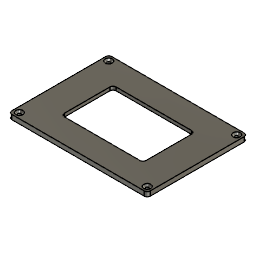
Lid V3.4 (Autodesk Fusion 360 design; units mm, degrees)
part number: 2026-01-29-14-58-12-979
Autodesk Fusion 360 part; units mm, degrees
note: some values were not read from the file. Set by a fixed rule: which sketch regions a step uses.
sketch "Sketch2" plane through (0, 0, 0) normal (0, 0, 1) x (1, 0, 0)
  line L0 (-48, 52) -> (124, 52)
  line L1 (128, 48) -> (128, -74)
  line L2 (124, -78) -> (-48, -78)
  line L3 (-52, -74) -> (-52, 48)
  circle A0 centre (-45, 45) radius 2.25
  line L4 (38, -78) -> (38, 52) construction
  line L5 (-52, -13) -> (128, -13) construction
  arc A1 (-48, 52) -> (-52, 48) centre (-48, 48) ccw
  circle A2 centre (121, 45) radius 2.25
  arc A3 (128, 48) -> (124, 52) centre (124, 48) ccw
  circle A4 centre (121, -71) radius 2.25
  arc A5 (124, -78) -> (128, -74) centre (124, -74) ccw
  circle A6 centre (-45, -71) radius 2.25
  arc A7 (-52, -74) -> (-48, -78) centre (-48, -74) ccw
  point P0 (-52, 52)
  point P1 (128, 52)
  dimension "d3" = 4.5
  dimension "d4" = 7
  dimension "d5" = 7
  dimension "d6" = 4
  dimension "d63" = 180
  dimension "d64" = 130
  constraint horizontal L0
  constraint vertical L1
  constraint horizontal L2
  constraint vertical L3
  constraint coincident L0 L4.end
  constraint coincident L3 L5.start
  constraint coincident P0 L0
  constraint coincident P0 L3
  constraint tangent L0 A1
  constraint tangent L3 A1
  constraint symmetric P0 L4 P1
  constraint symmetric A0 L4 A2
  constraint symmetric L4 L0.start L0.end
  constraint symmetric L4 L3.end L1.start
  constraint symmetric L4 A1 A3
  constraint coincident L1 L5.end
  constraint symmetric A0 L5 A6
  constraint symmetric L5 L0.start L2.end
  constraint symmetric L5 L3.end L3.start
  constraint symmetric L5 A1 A7
  constraint symmetric L5 L1.start L1.end
  constraint symmetric L5 L0.end L2.start
  constraint symmetric L5 A2 A4
  constraint symmetric L5 A3 A5
  constraint coincident L2 L4.start
  measures "d3" diameter of A0
  measures "d4" distance of L0 A0.centre
  measures "d5" distance of L3 A0.centre
  measures "d6" radius of A1
  measures "d63" distance of L1 L3
  measures "d64" distance of L0 L2
extrude "Extrude1" add sketch "Sketch2" along normal blind 6
sketch "Sketch3" plane through (0, 0, 0) normal (0, 0, -1) x (1, 0, 0)
  circle A0 centre (121, 71) radius 2.25
  circle A1 centre (-45, 71) radius 2.25
  circle A2 centre (-45, -45) radius 2.25
  circle A3 centre (121, -45) radius 2.25
  arc A4 (-52, -48) -> (-48, -52) centre (-48, -48) ccw
  line L0 (-48, -52) -> (124, -52)
  arc A5 (124, -52) -> (128, -48) centre (124, -48) ccw
  line L1 (128, -48) -> (128, 74)
  arc A6 (128, 74) -> (124, 78) centre (124, 74) ccw
  line L2 (124, 78) -> (-48, 78)
  arc A7 (-48, 78) -> (-52, 74) centre (-48, 74) ccw
  line L3 (-52, 74) -> (-52, -48)
  line L4 (38, 78) -> (38, -52) construction
  line L5 (128, 13) -> (-52, 13) construction
  line L6 (117.9494, -41.9494) -> (-41.9494, -41.9494) construction
  line L7 (-41.9494, -41.9494) -> (-41.9494, 67.9494) construction
  line L8 (-41.9494, 67.9494) -> (117.9494, 67.9494) construction
  line L9 (117.9494, 67.9494) -> (117.9494, -41.9494) construction
  line L10 (117.9494, -41.9494) -> (-41.9494, 67.9494) construction
  line L11 (-41.9494, -41.9494) -> (117.9494, 67.9494) construction
  line L12 (106.2459, -44.0839) -> (-30.2459, -44.0839)
  line L13 (-44.0839, -30.2459) -> (-44.0839, 56.2459)
  line L14 (-30.2459, 70.0839) -> (106.2459, 70.0839)
  line L15 (120.0839, 56.2459) -> (120.0839, -30.2459)
  line L16 (93.976, -25.9276) -> (-44.0839, 70.0839) construction
  line L17 (-38.2879, -33.8258) -> (83.9414, 41.199) construction
  line L18 (-39.8149, -30.2459) -> (-39.8149, 56.2459)
  line L19 (-30.2459, 65.8149) -> (106.2459, 65.8149)
  line L20 (115.8149, 56.2459) -> (115.8149, -30.2459)
  line L21 (103.0391, -31.1436) -> (-39.8149, 65.8149) construction
  line L22 (-35.6113, -30.989) -> (81.1607, 38.7921) construction
  arc A8 (-30.2459, 65.8149) -> (-39.8149, 56.2459) centre (-30.2459, 56.2459) ccw
  arc A9 (-30.2459, 70.0839) -> (-44.0839, 56.2459) centre (-30.2459, 56.2459) ccw
  arc A10 (115.8149, 56.2459) -> (106.2459, 65.8149) centre (106.2459, 56.2459) ccw
  arc A11 (120.0839, 56.2459) -> (106.2459, 70.0839) centre (106.2459, 56.2459) ccw
  arc A12 (-39.8149, -30.2459) -> (-30.2459, -39.8149) centre (-30.2459, -30.2459) ccw
  arc A13 (-44.0839, -30.2459) -> (-30.2459, -44.0839) centre (-30.2459, -30.2459) ccw
  arc A14 (106.2459, -39.8149) -> (115.8149, -30.2459) centre (106.2459, -30.2459) ccw
  arc A15 (106.2459, -44.0839) -> (120.0839, -30.2459) centre (106.2459, -30.2459) ccw
  line L23 (106.2459, -39.8149) -> (-30.2459, -39.8149)
  point P0 (38, 13)
  point P1 (38, 13)
  point P2 (38, 13)
  point P3 (38, 13)
  point P4 (38, 13)
  dimension "d25" = 159.8988
  dimension "d27" = 109.8988
  dimension "d28" = 2.1345
  dimension "d29" = 2.1345
  dimension "d30" = 2.1345
  dimension "d31" = 2.1345
  dimension "d44" = 9.569
  dimension "d45" = 13.838
  constraint midpoint L2 L4.start
  constraint midpoint L0 L4.end
  constraint midpoint L1 L5.start
  constraint midpoint L3 L5.end
  constraint midpoint L4 P4
  constraint coincident P4 P3
  constraint horizontal L6
  constraint perpendicular L6 L7
  constraint parallel L6 L8
  constraint parallel L7 L9
  constraint coincident L10 P4
  constraint coincident L11 P4
  constraint horizontal L12
  constraint perpendicular L12 L13
  constraint parallel L12 L14
  constraint parallel L13 L15
  constraint coincident L16 P4
  constraint coincident L17 P4
  constraint perpendicular L18 L23
  constraint parallel L19 L23
  constraint parallel L18 L20
  constraint coincident L21 P4
  constraint coincident L22 P4
  constraint coincident L21.end L19
  constraint coincident L21.end L18
  constraint tangent L19 A8
  constraint tangent L18 A8
  constraint coincident L16.end L14
  constraint coincident L16.end L13
  constraint tangent L14 A9
  constraint tangent L13 A9
  constraint symmetric L4 L19.start L19.end
  constraint symmetric L4 L18.end L20.start
  constraint symmetric L4 A8 A10
  constraint symmetric L4 L14.start L14.end
  constraint symmetric L4 L13.end L15.start
  constraint symmetric L4 A9 A11
  constraint symmetric L5 L19.start A12.end
  constraint symmetric L5 L18.end L18.start
  constraint symmetric L5 A8 A12
  constraint symmetric L5 L14.start L12.end
  constraint symmetric L5 L13.end L13.start
  constraint symmetric L5 A9 A13
  constraint symmetric L5 L19.end A14.start
  constraint symmetric L5 L20.start L20.end
  constraint symmetric L5 A10 A14
  constraint symmetric L5 L14.end L12.start
  constraint symmetric L5 L15.start L15.end
  constraint symmetric L5 A11 A15
  measures "d25" distance of L7.end L8.end
  measures "d27" distance of L6.end L7.end
  measures "d28" distance of L9 L15
  measures "d29" distance of L8 L14
  measures "d30" distance of L8 L19
  measures "d31" distance of L9 L20
  measures "d44" radius of A8
  measures "d45" radius of A9
extrude "Extrude4" add sketch "Sketch3" along normal blind 1.424 contours L12 L13 L14 L15 A9 A11 A13 A15
draft "Draft3" angle 10 neutral plane through (0, 0, -1.424) pull (0, 0, -1) 16 faces at (60.7486, -65.8149, -0.9493) (109.3756, -65.2886, -0.9493) (115.8149, -27.4153, -0.4747) (108.5019, 39.5452, -0.9493) (60.7486, 39.8149, -0.4747) (-38.5329, 35.0304, -0.9493) (-39.8149, -27.4153, -0.4747) (-32.5019, -65.5452, -0.9493) (-44.0839, 1.4153, -0.4747) (-35.389, 43.0927, -0.9493) (15.2514, 44.0839, -0.9493) (116.2609, 39.7952, -0.9493) (120.0839, 1.4153, -0.9493) (108.8648, -69.8338, -0.9493) (60.7486, -70.0839, -0.9493) (-44.0213, -57.5613, -0.4747)
sketch "Sketch5" plane through (0, 0, -1.424) normal (0, 0, -1) x (1, 0, 0)
  line L0 (-30.2459, 65.8149) -> (106.2459, 65.8149)
  line L1 (115.8149, 56.2459) -> (115.8149, -30.2459)
  line L2 (106.2459, -39.8149) -> (-30.2459, -39.8149)
  line L3 (-39.8149, -30.2459) -> (-39.8149, 56.2459)
  line L4 (106.2459, 70.0839) -> (-30.2459, 70.0839)
  line L5 (-44.0839, 56.2459) -> (-44.0839, -30.2459)
  line L6 (-30.2459, -44.0839) -> (106.2459, -44.0839)
  line L7 (120.0839, -30.2459) -> (120.0839, 56.2459)
  line L8 (38, 70.0839) -> (38, -44.0839) construction
  line L9 (120.0839, 13) -> (-44.0839, 13) construction
  line L10 (117.9494, -41.9494) -> (-41.9494, -41.9494) construction
  line L11 (-41.9494, -41.9494) -> (-41.9494, 67.9494) construction
  line L12 (-41.9494, 67.9494) -> (117.9494, 67.9494) construction
  line L13 (117.9494, 67.9494) -> (117.9494, -41.9494) construction
  line L14 (117.9494, -41.9494) -> (-41.9494, 67.9494) construction
  line L15 (-41.9494, -41.9494) -> (117.9494, 67.9494) construction
  line L16 (106.2459, -42.8839) -> (-30.2459, -42.8839)
  line L17 (-42.8839, -30.2459) -> (-42.8839, 56.2459)
  line L18 (-30.2459, 68.8839) -> (106.2459, 68.8839)
  line L19 (118.8839, 56.2459) -> (118.8839, -30.2459)
  line L20 (96.0985, -27.1411) -> (-42.8839, 68.8839) construction
  line L21 (-42.8839, -42.8839) -> (96.0985, 53.1411) construction
  line L22 (106.2459, -41.0149) -> (-30.2459, -41.0149)
  line L23 (-41.0149, -30.2459) -> (-41.0149, 56.2459)
  line L24 (117.0149, 56.2459) -> (117.0149, -30.2459)
  line L25 (95.1479, -26.0666) -> (-41.0149, 67.0149) construction
  line L26 (-41.0149, -41.0149) -> (95.1479, 52.0666) construction
  arc A0 (115.8149, 56.2459) -> (106.2459, 65.8149) centre (106.2459, 56.2459) ccw
  arc A1 (106.2459, -39.8149) -> (115.8149, -30.2459) centre (106.2459, -30.2459) ccw
  arc A2 (-39.8149, -30.2459) -> (-30.2459, -39.8149) centre (-30.2459, -30.2459) ccw
  arc A3 (-30.2459, 65.8149) -> (-39.8149, 56.2459) centre (-30.2459, 56.2459) ccw
  arc A4 (-44.0839, -30.2459) -> (-30.2459, -44.0839) centre (-30.2459, -30.2459) ccw
  arc A5 (106.2459, -44.0839) -> (120.0839, -30.2459) centre (106.2459, -30.2459) ccw
  arc A6 (120.0839, 56.2459) -> (106.2459, 70.0839) centre (106.2459, 56.2459) ccw
  arc A7 (-30.2459, 70.0839) -> (-44.0839, 56.2459) centre (-30.2459, 56.2459) ccw
  arc A8 (-30.2459, 67.0149) -> (-41.0149, 56.2459) centre (-30.2459, 56.2459) ccw
  arc A9 (-30.2459, 68.8839) -> (-42.8839, 56.2459) centre (-30.2459, 56.2459) ccw
  arc A10 (117.0149, 56.2459) -> (106.2459, 67.0149) centre (106.2459, 56.2459) ccw
  arc A11 (118.8839, 56.2459) -> (106.2459, 68.8839) centre (106.2459, 56.2459) ccw
  line L27 (-30.2459, 67.0149) -> (106.2459, 67.0149)
  arc A12 (106.2459, -41.0149) -> (117.0149, -30.2459) centre (106.2459, -30.2459) ccw
  arc A13 (106.2459, -42.8839) -> (118.8839, -30.2459) centre (106.2459, -30.2459) ccw
  arc A14 (-41.0149, -30.2459) -> (-30.2459, -41.0149) centre (-30.2459, -30.2459) ccw
  arc A15 (-42.8839, -30.2459) -> (-30.2459, -42.8839) centre (-30.2459, -30.2459) ccw
  point P0 (38, 13)
  point P1 (38, 13)
  point P2 (38, 13)
  dimension "d36" = 159.8988
  dimension "d37" = 109.8988
  dimension "d38" = 0.9345
  dimension "d39" = 0.9345
  dimension "d40" = 0.9345
  dimension "d41" = 0.9345
  dimension "d50" = 10.769
  dimension "d51" = 12.638
  constraint midpoint L4 L8.start
  constraint midpoint L6 L8.end
  constraint midpoint L7 L9.start
  constraint midpoint L5 L9.end
  constraint horizontal L10
  constraint perpendicular L10 L11
  constraint parallel L10 L12
  constraint parallel L11 L13
  constraint coincident L14 P2
  constraint coincident L15 P2
  constraint midpoint L8 P2
  constraint horizontal L16
  constraint perpendicular L16 L17
  constraint parallel L16 L18
  constraint parallel L17 L19
  constraint coincident L20 P2
  constraint coincident L21 P2
  constraint coincident P2 P1
  constraint horizontal L22
  constraint perpendicular L22 L23
  constraint parallel L22 L27
  constraint parallel L23 L24
  constraint coincident L25 P2
  constraint coincident L26 P2
  constraint coincident L26.start L23
  constraint coincident L26.start L22
  constraint coincident L21.start L17
  constraint coincident L21.start L16
  constraint coincident L25.end L27
  constraint coincident L25.end L23
  constraint tangent A8 L27
  constraint tangent L23 A8
  constraint coincident L20.end L18
  constraint coincident L20.end L17
  constraint tangent L18 A9
  constraint tangent L17 A9
  constraint symmetric L8 A8.start A10.end
  constraint symmetric L8 L23.end L24.start
  constraint symmetric L8 A8 A10
  constraint symmetric L8 L18.start L18.end
  constraint symmetric L8 L17.end L19.start
  constraint symmetric L8 A9 A11
  constraint symmetric L9 A10.end L22.start
  constraint symmetric L9 L24.start L24.end
  constraint symmetric L9 A10 A12
  constraint symmetric L9 L18.end L16.start
  constraint symmetric L9 L19.start L19.end
  constraint symmetric L9 A11 A13
  constraint symmetric L9 A8.start L22.end
  constraint symmetric L9 L23.end L23.start
  constraint symmetric L9 A8 A14
  constraint symmetric L9 L18.start L16.end
  constraint symmetric L9 L17.end L17.start
  constraint symmetric L9 A9 A15
  constraint coincident L23.start A14.start
  constraint coincident L17.start A15.start
  constraint coincident L22.end A14.end
  constraint coincident L16.end A15.end
  measures "d36" distance of L11.end L12.end
  measures "d37" distance of L10.end L11.end
  measures "d38" distance of L13 L19
  measures "d39" distance of L13 L24
  measures "d40" distance of L10 L16
  measures "d41" distance of L10 L22
  measures "d50" radius of A8
  measures "d51" radius of A9
extrude "Extrude6" cut sketch "Sketch5" against normal blind 1.424 contours L16 L17 L18 L19 A9 A11 A13 A15
extrude "Extrude7" cut 1 faces at (15.2514, -30.5213, 0) along direction (0, 0, 1) blind 0.5
sketch "Sketch6" plane through (0, 0, 0.5) normal (0, 0, -1) x (1, 0, 0)
  line L0 (106.2459, 65.5638) -> (-30.2459, 65.5638)
  arc A0 (-30.2459, 65.5638) -> (-39.5638, 56.2459) centre (-30.2459, 56.2459) ccw
  line L1 (-39.5638, 56.2459) -> (-39.5638, -30.2459)
  arc A1 (-39.5638, -30.2459) -> (-30.2459, -39.5638) centre (-30.2459, -30.2459) ccw
  line L2 (-30.2459, -39.5638) -> (106.2459, -39.5638)
  arc A2 (106.2459, -39.5638) -> (115.5638, -30.2459) centre (106.2459, -30.2459) ccw
  line L3 (115.5638, -30.2459) -> (115.5638, 56.2459)
  arc A3 (115.5638, 56.2459) -> (106.2459, 65.5638) centre (106.2459, 56.2459) ccw
  line L4 (38, 65.5638) -> (38, -39.5638) construction
  line L5 (-39.5638, 13) -> (115.5638, 13) construction
  line L6 (92, -25.5) -> (-16, -25.5)
  line L7 (-20, -21.5) -> (-20, 47.5)
  line L8 (-16, 51.5) -> (92, 51.5)
  line L9 (96, 47.5) -> (96, -21.5)
  line L10 (96, -25.5) -> (-20, 51.5) construction
  line L11 (-20, -25.5) -> (96, 51.5) construction
  arc A4 (-16, 51.5) -> (-20, 47.5) centre (-16, 47.5) ccw
  arc A5 (96, 47.5) -> (92, 51.5) centre (92, 47.5) ccw
  arc A6 (92, -25.5) -> (96, -21.5) centre (92, -21.5) ccw
  arc A7 (-20, -21.5) -> (-16, -25.5) centre (-16, -21.5) ccw
  point P0 (38, 13)
  dimension "d58" = 116
  dimension "d59" = 77
  dimension "d68" = 4
  dimension "d69" = 4
  dimension "d70" = 4
  dimension "d71" = 4
  constraint midpoint L0 L4.start
  constraint midpoint L2 L4.end
  constraint midpoint L1 L5.start
  constraint midpoint L3 L5.end
  constraint horizontal L6
  constraint perpendicular L6 L7
  constraint parallel L6 L8
  constraint parallel L7 L9
  constraint coincident L10 P0
  constraint coincident L11 P0
  constraint midpoint L5 P0
  constraint coincident L10.end L8
  constraint coincident L10.end L7
  constraint tangent L8 A4
  constraint tangent L7 A4
  constraint coincident L11.end L8
  constraint coincident L11.end L9
  constraint tangent L8 A5
  constraint tangent L9 A5
  constraint coincident L10.start L9
  constraint coincident L10.start L6
  constraint tangent L9 A6
  constraint tangent L6 A6
  constraint coincident L11.start L7
  constraint coincident L11.start L6
  constraint tangent L7 A7
  constraint tangent L6 A7
  measures "d58" distance of L10.end L11.end
  measures "d59" distance of L11.start L10.end
  measures "d68" radius of A4
  measures "d69" radius of A5
  measures "d70" radius of A6
  measures "d71" radius of A7
extrude "Extrude8" cut sketch "Sketch6" against normal blind 1.1 contours L6 L7 L8 L9 A4 A5 A6 A7
sketch "Sketch7" plane through (0, 0, 1.6) normal (0, 0, -1) x (1, 0, 0)
  line L0 (92, 51.5) -> (-16, 51.5)
  line L1 (-20, 47.5) -> (-20, -21.5)
  line L2 (-16, -25.5) -> (92, -25.5)
  line L3 (96, -21.5) -> (96, 47.5)
  line L4 (38, 51.5) -> (38, -25.5) construction
  line L5 (96, 13) -> (-20, 13) construction
  line L6 (87, -20.5) -> (-11, -20.5)
  line L7 (-15, -16.5) -> (-15, 42.5)
  line L8 (-11, 46.5) -> (87, 46.5)
  line L9 (91, 42.5) -> (91, -16.5)
  line L10 (91, -20.5) -> (-15, 46.5) construction
  line L11 (-15, -20.5) -> (91, 46.5) construction
  arc A0 (-16, 51.5) -> (-20, 47.5) centre (-16, 47.5) ccw
  arc A1 (-20, -21.5) -> (-16, -25.5) centre (-16, -21.5) ccw
  arc A2 (92, -25.5) -> (96, -21.5) centre (92, -21.5) ccw
  arc A3 (96, 47.5) -> (92, 51.5) centre (92, 47.5) ccw
  arc A4 (-11, 46.5) -> (-15, 42.5) centre (-11, 42.5) ccw
  arc A5 (91, 42.5) -> (87, 46.5) centre (87, 42.5) ccw
  arc A6 (87, -20.5) -> (91, -16.5) centre (87, -16.5) ccw
  arc A7 (-15, -16.5) -> (-11, -20.5) centre (-11, -16.5) ccw
  point P0 (38, 13)
  dimension "d62" = 106
  dimension "d65" = 67
  dimension "d72" = 4
  dimension "d73" = 4
  dimension "d74" = 4
  dimension "d75" = 4
  constraint midpoint L0 L4.start
  constraint midpoint L2 L4.end
  constraint midpoint L3 L5.start
  constraint midpoint L1 L5.end
  constraint horizontal L6
  constraint perpendicular L6 L7
  constraint parallel L6 L8
  constraint parallel L7 L9
  constraint coincident L10 P0
  constraint coincident L11 P0
  constraint midpoint L4 P0
  constraint coincident L10.end L8
  constraint coincident L10.end L7
  constraint tangent L8 A4
  constraint tangent L7 A4
  constraint coincident L11.end L9
  constraint coincident L11.end L8
  constraint tangent L9 A5
  constraint tangent L8 A5
  constraint coincident L10.start L9
  constraint coincident L10.start L6
  constraint tangent L9 A6
  constraint tangent L6 A6
  constraint coincident L11.start L6
  constraint coincident L11.start L7
  constraint tangent L6 A7
  constraint tangent L7 A7
  measures "d62" distance of L10.end L11.end
  measures "d65" distance of L11.start L10.end
  measures "d72" radius of A4
  measures "d73" radius of A5
  measures "d74" radius of A6
  measures "d75" radius of A7
extrude "Extrude9" cut sketch "Sketch7" against normal blind 8.4 contours L6 L7 L8 L9 A4 A5 A6 A7
sketch "Sketch9" plane through (0, 0, 6) normal (0, 0, 1) x (-1, 0, 0)
  line L0 (15, 42.5) -> (15, -16.5)
  arc A0 (11, -20.5) -> (15, -16.5) centre (11, -16.5) ccw
  line L1 (11, -20.5) -> (-87, -20.5)
  arc A1 (-91, -16.5) -> (-87, -20.5) centre (-87, -16.5) ccw
  line L2 (-91, -16.5) -> (-91, 42.5)
  arc A2 (-87, 46.5) -> (-91, 42.5) centre (-87, 42.5) ccw
  line L3 (-87, 46.5) -> (11, 46.5)
  arc A3 (15, 42.5) -> (11, 46.5) centre (11, 42.5) ccw
  circle A4 centre (-121, 71) radius 2.25
  circle A5 centre (-121, -45) radius 2.25
  circle A6 centre (45, 71) radius 2.25
  circle A7 centre (45, -45) radius 2.25
  arc A8 (48, -52) -> (52, -48) centre (48, -48) ccw
  line L4 (52, -48) -> (52, 74)
  arc A9 (52, 74) -> (48, 78) centre (48, 74) ccw
  line L5 (48, 78) -> (-124, 78)
  arc A10 (-124, 78) -> (-128, 74) centre (-124, 74) ccw
  line L6 (-128, 74) -> (-128, -48)
  arc A11 (-128, -48) -> (-124, -52) centre (-124, -48) ccw
  line L7 (-124, -52) -> (48, -52)
  line L8 (45, -47.25) -> (45, -42.75) construction
  line L9 (42.75, -45) -> (47.25, -45) construction
  circle A12 centre (45, -45) radius 4
  line L10 (-38, -52) -> (-38, 78) construction
  line L11 (-128, 13) -> (52, 13) construction
  circle A13 centre (-121, -45) radius 4
  circle A14 centre (45, 71) radius 4
  circle A15 centre (-121, 71) radius 4
  dimension "d91" = 8
  constraint coincident A7 L8.start
  constraint coincident A7 L8.end
  constraint vertical L8
  constraint coincident A7 L9.start
  constraint coincident A7 L9.end
  constraint perpendicular L8 L9
  constraint concentric A7 A12
  constraint midpoint L7 L10.start
  constraint midpoint L5 L10.end
  constraint midpoint L6 L11.start
  constraint midpoint L4 L11.end
  constraint symmetric A12 L10 A13
  constraint symmetric A12 L11 A14
  constraint symmetric L11 A13 A15
  measures "d91" diameter of A12
sketch "Sketch10" plane through (0, 0, 0.5) normal (0, 0, -1) x (1, 0, 0)
  line L0 (-20, -21.5) -> (-20, 47.5)
  arc A0 (-16, 51.5) -> (-20, 47.5) centre (-16, 47.5) ccw
  line L1 (-16, 51.5) -> (92, 51.5)
  arc A1 (96, 47.5) -> (92, 51.5) centre (92, 47.5) ccw
  line L2 (96, 47.5) -> (96, -21.5)
  arc A2 (92, -25.5) -> (96, -21.5) centre (92, -21.5) ccw
  line L3 (92, -25.5) -> (-16, -25.5)
  arc A3 (-20, -21.5) -> (-16, -25.5) centre (-16, -21.5) ccw
  line L4 (106.2459, 65.5638) -> (-30.2459, 65.5638)
  arc A4 (-30.2459, 65.5638) -> (-39.5638, 56.2459) centre (-30.2459, 56.2459) ccw
  line L5 (-39.5638, 56.2459) -> (-39.5638, -30.2459)
  arc A5 (-39.5638, -30.2459) -> (-30.2459, -39.5638) centre (-30.2459, -30.2459) ccw
  line L6 (-30.2459, -39.5638) -> (106.2459, -39.5638)
  arc A6 (106.2459, -39.5638) -> (115.5638, -30.2459) centre (106.2459, -30.2459) ccw
  line L7 (115.5638, -30.2459) -> (115.5638, 56.2459)
  arc A7 (115.5638, 56.2459) -> (106.2459, 65.5638) centre (106.2459, 56.2459) ccw
  line L8 (38, 65.5638) -> (38, -39.5638) construction
  line L9 (115.5638, 13) -> (-39.5638, 13) construction
  line L10 (38, 13) -> (-24.24, 13) construction
  line L11 (-23.09, 11) -> (-25.39, 11)
  line L12 (-25.39, 11) -> (-25.39, 15)
  line L13 (-25.39, 15) -> (-23.09, 15)
  line L14 (-23.09, 15) -> (-23.09, 11)
  line L15 (-23.09, 11) -> (-25.39, 15) construction
  line L16 (-25.39, 11) -> (-23.09, 15) construction
  line L17 (38, 13) -> (38, 54) construction
  line L18 (40, 52.85) -> (36, 52.85)
  line L19 (36, 52.85) -> (36, 55.15)
  line L20 (36, 55.15) -> (40, 55.15)
  line L21 (40, 55.15) -> (40, 52.85)
  line L22 (40, 52.85) -> (36, 55.15) construction
  line L23 (36, 52.85) -> (40, 55.15) construction
  line L24 (99.09, 15) -> (99.09, 11)
  line L25 (101.39, 15) -> (99.09, 15)
  line L26 (101.39, 11) -> (101.39, 15)
  line L27 (99.09, 11) -> (101.39, 11)
  line L28 (40, -26.85) -> (36, -26.85)
  line L29 (40, -29.15) -> (40, -26.85)
  line L30 (36, -29.15) -> (40, -29.15)
  line L31 (36, -26.85) -> (36, -29.15)
  point P0 (-24.24, 13)
  point P1 (38, 54)
  dimension "d97" = 62.24
  dimension "d98" = 2.3
  dimension "d99" = 4
  dimension "d100" = 41
  dimension "d101" = 2.3
  dimension "d102" = 4
  constraint midpoint L4 L8.start
  constraint midpoint L6 L8.end
  constraint midpoint L7 L9.start
  constraint midpoint L5 L9.end
  constraint midpoint L9 L10.start
  constraint perpendicular L8 L10
  constraint horizontal L11
  constraint perpendicular L11 L12
  constraint parallel L11 L13
  constraint parallel L12 L14
  constraint coincident L15 P0
  constraint coincident L16 P0
  constraint coincident P0 L10.end
  constraint perpendicular L9 L17
  constraint horizontal L18
  constraint perpendicular L18 L19
  constraint parallel L18 L20
  constraint parallel L19 L21
  constraint coincident L22 P1
  constraint coincident L23 P1
  constraint coincident P1 L17.end
  constraint symmetric L8 L11.start L24.end
  constraint symmetric L8 L11.end L26.start
  constraint symmetric L8 L12.end L25.start
  constraint symmetric L8 L13.end L24.start
  constraint symmetric L9 L18.start L28.start
  constraint symmetric L9 L18.end L28.end
  constraint symmetric L9 L19.end L30.start
  constraint symmetric L9 L20.end L29.start
  measures "d97" distance of L10.start P0
  measures "d98" distance of L12.end L13.end
  measures "d99" distance of L11.end L12.end
  measures "d100" distance of L10.start P1
  measures "d101" distance of L18.start L20.end
  measures "d102" distance of L19.end L20.end
extrude "Extrude12" add sketch "Sketch10" along normal blind 4.2 contours L11 L12 L13 L14 | L18 L19 L20 L21 | L24 L25 L26 L27 | L28 L29 L30 L31
chamfer "Chamfer2" distance 2.4 angle 45 4 edges at (-47.0977, 45.8136, 6) (118.9023, 45.8136, 6) (118.9023, -70.1864, 6) (-47.0977, -70.1864, 6) measured on face at (111.574, -3.1667, 6) measured on face at (111.574, -3.1667, 6) measured on face at (111.574, -3.1667, 6) measured on face at (111.574, -3.1667, 6)
equation "d3 = Bolt_Diam + 0.5 mm"
equation "ORingDiameter = 1.78 mm" comment "Diamter of the O ring"
equation "ORingInnerDiameter = 170 mm" comment "Inner diamter of the o ring bore"
equation "d25 = ( ORingPerimeter - 100 mm ) / 4 + 50 mm"
equation "ORingPerimeter = 2 * 3.1412 * ( ( ORingInnerDiameter / 2 ) + ORingDiameter / 2 )"
equation "d27 = ( ORingPerimeter - 100 mm ) / 4"
equation "d28 = ( ( ORingDiameter * 1.05 ) / 2 ) + 1.2 mm"
equation "d29 = ( ( ORingDiameter * 1.05 ) / 2 ) + 1.2 mm"
equation "d30 = ( ( ORingDiameter * 1.05 ) / 2 ) + 1.2 mm"
equation "d31 = ( ( ORingDiameter * 1.05 ) / 2 ) + 1.2 mm"
equation "d32 = ORingDiameter * 0.8"
equation "d36 = ( ORingPerimeter - 100 mm ) / 4 + 50 mm"
equation "d37 = ( ORingPerimeter - 100 mm ) / 4"
equation "d38 = ( ORingDiameter * 1.05 ) / 2"
equation "d39 = ( ORingDiameter * 1.05 ) / 2"
equation "d40 = ( ORingDiameter * 1.05 ) / 2"
equation "d41 = ( ORingDiameter * 1.05 ) / 2"
equation "d44 = ( ORingDiameter ) * 6 + ORingDiameter * 0.05 - 1.2 mm"
equation "d45 = ( ORingDiameter ) * 6 + ( ORingDiameter * 1.1 ) + 1.2 mm"
equation "d50 = ( ORingDiameter ) * 6 + ORingDiameter * 0.05 - 0.0 mm"
equation "d51 = ( ORingDiameter ) * 6 + ORingDiameter * 1.1 + 0 mm"
equation "d52 = -( ORingDiameter * 0.8 )"
equation "PanelWidth = 77 mm"
equation "PanelLength = 116 mm"
equation "d58 = PanelLength"
equation "d59 = PanelWidth"
equation "d62 = PanelLength - 10 mm"
equation "d65 = PanelWidth - 10 mm"
equation "d91 = Bolt_Head_Diam"
equation "Bolt_Diam = 4 mm" comment "Diameter of the bolt"
equation "Bolt_Head_Height = 2.3 mm" comment "Height of th ebolt head"
equation "Bolt_Head_Diam = 8 mm" comment "Diamter of the bolt head"
equation "d106 = Bolt_Head_Height + 0.1 mm"
